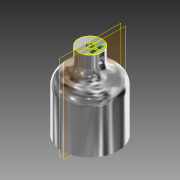
# Autodesk Inventor part: support shaft end
Saved by Autodesk Inventor 2013 (Build 170138000, 138)
## iProperties
Created: 2015-01-06
Part Number: support shaft end
Material: Generic
Document SubType Name: Modeling
Designer: Nico
Density: 1 g/cm^3
Author: Nico
Autodesk Inventor part; units mm, degrees
ref_plane "YZ Plane" through (0, 0, 0) normal (1, 0, 0) x (0, 1, 0)
sketch "Sketch1" plane through (0, 0, 0) normal (0, 0, 1) x (1, 0, 0)
  circle A0 centre (0, 0) radius 12
  circle A1 centre (0, 0) radius 1.5
  dimension "d0" = 24
  dimension "d2" = 3
  constraints: 2 centre point, 2 coincident
  measures "d0" diameter of A0
  measures "d2" diameter of A1
extrude "Extrusion1" add sketch "Sketch1" along normal blind 3
sketch "Sketch2" plane through (0, 0, 3) normal (0, 0, 1) x (1, 0, 0)
  circle A0 centre (0, 0) radius 1.5 projected
  circle A1 centre (0, 0) radius 12 projected
  circle A2 centre (0, 0) radius 5
  dimension "d5" = 10
  constraints: 1 centre point, 1 coincident
  measures "d5" diameter of A2
extrude "Extrusion2" add sketch "Sketch2" along normal blind 10 contours A2
sketch "Sketch14" plane through (0, 0, 0) normal (0, 0, -1) x (-1, 0, 0)
  circle A0 centre (0, 0) radius 1.5 projected
  circle A1 centre (0, 0) radius 12 projected
extrude "Extrusion11" add sketch "Sketch14" along normal blind 20
ref_plane "Work Plane6" through (0, 0, 8) normal (0, 0, 1) x (1, 0, 0)
sketch "Sketch15" plane through (0, 0, 8) normal (0, 0, 1) x (1, 0, 0)
  line L0 (0, -4.8919) -> (0, 6.5751)
  point P0 (0, 0)
  constraints: 2 end point, 1 vertical
ref_plane "Work Plane7" through (0, -4.8919, 8) normal (1, 0, 0) x (0, 1, 0)
fillet "Fillet3" radius 5 1 edges at (-5, 0, 3)
fillet "Fillet4" radius 5 1 edges at (-12, 0, 3)
sketch "Sketch17" plane through (0, 0, 13) normal (0, 0, 1) x (1, 0, 0)
  circle A0 centre (0, 0) radius 1.5 projected
  circle A1 centre (0, 0) radius 5 projected
  line L0 (0, -5) -> (0, 5)
  constraints: 2 end point, 2 point on circle, 1 vertical
ref_plane "Work Plane8" through (0, -5, 13) normal (1, 0, 0) x (0, 1, 0)
sketch "Sketch18" plane through (0, -5, 13) normal (1, 0, 0) x (0, 1, 0)
  circle A0 centre (5, -3) radius 1.3323
  line L0 (10, 0) -> (0, 0) projected
  point P0 (5, -13)
  dimension "d88" = 3
  constraints: 1 centre point
  measures "d88" distance from line of L0 A0.centre
extrude "Extrusion13" cut sketch "Sketch18" along normal blind 10
sketch "Sketch19" plane through (0, 0, 13) normal (0, 0, 1) x (1, 0, 0)
  circle A0 centre (0, 0) radius 1.5 projected
  line L0 (2, -2.75) -> (3.6, -2.75)
  line L1 (3.6, -2.75) -> (3.6, 2.75)
  line L2 (3.6, 2.75) -> (2, 2.75)
  line L3 (2, 2.75) -> (2, -2.75)
  dimension "d91" = 5.5
  dimension "d93" = 2.75
  dimension "d94" = 1.6
  dimension "d95" = 2
  constraints: 8 end point, 2 parallel, 1 horizontal, 1 perpendicular
  measures "d91" distance between parallel lines of L0 L2
  measures "d93" distance from line of L2 A0.centre
  measures "d94" distance between parallel lines of L1 L3
  measures "d95" distance from line of L3 A0.centre
ref_plane "Work Plane9" through (2, 2.75, 13) normal (1, 0, 0) x (0, -1, 0)
sketch "Sketch20" plane through (2, 2.75, 13) normal (1, 0, 0) x (0, -1, 0)
  line L0 (2.75, 6.1546) -> (5.5, 4.5669)
  line L1 (5.5, 4.5669) -> (5.5, 1.3914)
  line L2 (5.5, 1.3914) -> (2.75, -0.1963)
  line L3 (2.75, -0.1963) -> (0, 1.3914)
  line L4 (0, 1.3914) -> (0, 4.5669)
  line L5 (0, 4.5669) -> (2.75, 6.1546)
  point P0 (2.75, 13)
  point P1 (2.75, 2.9792)
  dimension "d97" = 5.5
  constraints: 12 end point, 13 other
  measures "d97" distance between parallel lines of L1 L4
extrude "Extrusion14" cut sketch "Sketch20" along normal blind 1.6
sketch "Sketch21" plane through (0, 0, 13) normal (0, 0, 1) x (1, 0, 0)
  line L0 (2, 0.34) -> (3.6, 0.34) projected
  line L1 (3.6, 0.34) -> (3.6, -0.34) projected
  line L2 (3.6, -0.34) -> (2, -0.34) projected
  line L3 (2, -0.34) -> (2, 0.34) projected
  circle A0 centre (0, 0) radius 1.5 projected
  circle A1 centre (0, 0) radius 5 projected
  line L4 (2, -2.7571) -> (3.6, -2.7571)
  line L5 (3.6, -2.7571) -> (3.6, 2.7571)
  line L6 (3.6, 2.7571) -> (2, 2.7571)
  line L7 (2, 2.7571) -> (2, -2.7571)
  constraints: 8 end point, 2 parallel, 1 horizontal, 1 perpendicular
extrude "Extrusion15" cut sketch "Sketch19" against normal blind 3 contours L3 L2 L1 L0
body "Solid1"
